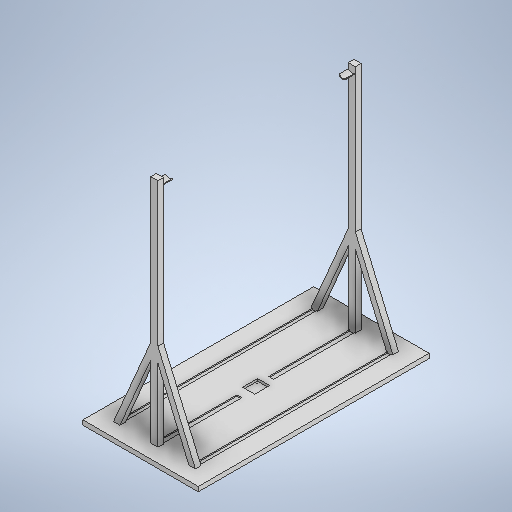
# Autodesk Inventor part: Structure_provisional
Saved by Autodesk Inventor 2025.1 (Build 291241020, 241B)
## iProperties
Created: 2025-09-05
Part Number: Structure_provisional
Material: Genérico
Document SubType Name: Modeling
Designer: Yo
Density: 1 g/cm^3
Appearance: Valor por defecto
Author: Yo
Autodesk Inventor part; units mm, degrees
ref_plane "YZ Plane" through (0, 0, 0) normal (1, 0, 0) x (0, 1, 0)
ref_plane "XZ Plane" through (0, 0, 0) normal (0, 1, 0) x (-1, 0, 0)
sketch "Boceto1" plane through (0, 0, 0) normal (0, 1, 0) x (-1, 0, 0)
  line L0 (0, 0) -> (0, -500) construction
  line L1 (0, -500) -> (500, -500) construction
  line L2 (500, -500) -> (500, 500) construction
  line L3 (500, 500) -> (0, 500) construction
  line L4 (0, 500) -> (0, 0) construction
  line L5 (500, 500) -> (0, 500)
  line L6 (0, 500) -> (0, -500)
  line L7 (0, -500) -> (500, -500)
  line L8 (500, -500) -> (500, 500)
  dimension "d0" = 500
  dimension "d1" = 500
  dimension "d2" = 1000
  constraints: 18 end point, 4 perpendicular, 3 equal length, 1 horizontal, 1 point on line, 1 vertical
  measures "d0" distance of L0.start L0.end
  measures "d1" distance of L0.end L1.end
  measures "d2" distance of L1.end L2.end
extrude "Extrusión1" add sketch "Boceto1" along normal blind 20
sketch "Boceto2" plane through (0, 20, 0) normal (0, 1, 0) x (1, 0, 0)
  line L0 (0, 500) -> (-500, 500) construction
  line L1 (-250, 500) -> (-250, -500) construction
  line L2 (-500, -500) -> (0, -500) construction
  line L3 (-265.9292, 440.1456) -> (-234.905, 440.1456)
  line L4 (-234.905, 440.1456) -> (-234.905, 415.7448)
  line L5 (-234.905, 415.7448) -> (-265.9292, 415.7448)
  line L6 (-265.9292, 415.7448) -> (-265.9292, 440.1456)
  point P0 (0, 0)
  constraints: 10 end point, 2 midpoint, 2 parallel, 1 horizontal, 1 perpendicular
extrude "Extrusión2" add sketch "Boceto2" along normal blind 1000
mirror "Simetría1" about plane through (0, 0, 0) normal (0, 0, 1) of "Extrusión2"
sketch "Boceto4" plane through (-265.9292, 20, 440.1456) normal (0, 0, 1) x (1, 0, 0)
  line L0 (31.0242, 0) -> (31.0242, 1000) construction
  line L1 (31.0242, 379.2693) -> (193.3148, 0) construction
  line L2 (31.0242, 314.0177) -> (165.3935, 0) construction
  line L3 (-234.0708, 0) -> (265.9292, 0) construction
  line L4 (31.0242, 379.2693) -> (193.3148, 0)
  line L5 (165.3935, 0) -> (31.0242, 314.0177)
  line L6 (31.0242, 379.2693) -> (31.0242, 314.0177)
  line L7 (165.3935, 0) -> (193.3148, 0)
  point P0 (265.9292, -20)
  constraints: 12 end point, 4 point on line, 3 collinear, 1 parallel
extrude "Extrusión3" add sketch "Boceto4" against normal up to surface (24.4008 mm away)
ref_plane "Plano de trabajo1" through (-250, 0, 500) normal (1, 0, 0) x (0, 0, -1)
mirror "Simetría2" about plane through (-250, 0, 500) normal (1, 0, 0) of "Extrusión3"
mirror "Simetría3" about plane through (0, 0, 0) normal (0, 0, 1) of "Extrusión3", "Simetría2"
sketch "Boceto5" plane through (0, 20, 0) normal (0, 1, 0) x (1, 0, 0)
  line L0 (-72.6144, 415.7448) -> (-234.905, 415.7448) construction
  line L1 (-78.0914, 415.7448) -> (-78.0914, 405.899) construction
  line L2 (-95.8718, 415.7448) -> (-95.8718, 405.899) construction
  line L3 (-78.0914, 415.7448) -> (-95.8718, 415.7448)
  line L4 (-95.8718, 0) -> (-95.8718, 415.7448)
  line L5 (-78.0914, 415.7448) -> (-78.0914, 0)
  line L6 (-78.0914, 0) -> (-78.0914, -415.7448)
  line L7 (-100.5357, -415.7448) -> (-72.6144, -415.7448) projected
  line L8 (-95.8718, 0) -> (-95.8718, -415.7448)
  line L9 (-78.0914, -415.7448) -> (-95.8718, -415.7448)
  point P0 (0, 0)
  constraints: 16 end point, 8 point on line, 2 collinear, 2 perpendicular, 1 vertical
extrude "Extrusión4" cut sketch "Boceto5" against normal blind 5
mirror "Simetría4" about plane through (-250, 0, 500) normal (1, 0, 0) of "Extrusión4"
sketch "Boceto6" plane through (0, 20, 0) normal (0, 1, 0) x (1, 0, 0)
  line L0 (-265.9292, 415.7448) -> (-234.905, 415.7448) construction
  line L1 (-239.0903, 415.7448) -> (-239.0903, 391.5107) construction
  line L2 (-260.3339, 415.7448) -> (-260.3339, 390.2687) construction
  line L3 (-265.9292, -415.7448) -> (-234.905, -415.7448) construction
  line L4 (-239.0903, 415.7448) -> (-260.3339, 415.7448) construction
  line L5 (-260.3339, -415.7448) -> (-239.0903, -415.7448) construction
  line L6 (-239.0903, -415.7448) -> (-260.3339, -415.7448)
  line L7 (-239.0903, 415.7448) -> (-260.3339, 415.7448)
  line L8 (-239.0903, 65.2159) -> (-260.3339, 65.2159)
  line L9 (-239.0903, -72.6288) -> (-260.3339, -72.6288)
  line L10 (-239.0903, -415.7448) -> (-239.0903, -72.6288)
  line L11 (-239.0903, 65.2159) -> (-239.0903, 415.7448)
  line L12 (-260.3339, 415.7448) -> (-260.3339, 65.2159)
  line L13 (-260.3339, -72.6288) -> (-260.3339, -415.7448)
  point P0 (0, 0)
  constraints: 24 end point, 6 perpendicular, 5 parallel, 3 point on line, 2 horizontal, 2 vertical, 1 collinear
extrude "Extrusión5" cut sketch "Boceto6" against normal blind 5
sketch "Boceto7" plane through (0, 20, 0) normal (0, 1, 0) x (1, 0, 0)
  line L0 (-224.1946, 33.7447) -> (-276.8566, 33.7447)
  line L1 (-276.8566, 33.7447) -> (-276.8566, -31.5828)
  line L2 (-276.8566, -31.5828) -> (-224.1946, -31.5828)
  line L3 (-224.1946, -31.5828) -> (-224.1946, 33.7447)
  point P0 (0, 0)
  constraints: 8 end point, 2 parallel, 1 horizontal, 1 perpendicular
extrude "Extrusión6" cut sketch "Boceto7" against normal blind 10
sketch "Boceto8" plane through (0, 10, 0) normal (0, 1, 0) x (1, 0, 0)
  point P0 (0, 0)
  point P1 (-230.6615, -24.5924)
hole "Agujero1" at (-230.6615, 10, 24.5924) direction (0, -1, 0) diameter 3 end through all
mirror "Simetría5" about plane through (-250, 0, 500) normal (1, 0, 0) of "Agujero1"
mirror "Simetría6" about plane through (0, 0, 0) normal (0, 0, 1) of "Agujero1", "Simetría5"
sketch "Boceto9" plane through (-265.9292, 397.3198, -415.7448) normal (0, 0, 1) x (1, 0, 0)
  line L0 (0, 0) -> (0, 622.6802) projected
  line L1 (31.0242, 1.9495) -> (31.0242, 622.6802) projected
  arc A0 (0, 595.7054) -> (31.0242, 595.8449) centre (15.4643, 606.4176) ccw
  line L2 (0, 595.7054) -> (0, 599.8174)
  line L3 (31.0242, 595.8449) -> (31.0242, 599.8174)
  arc A1 (0, 599.8174) -> (31.0242, 599.8174) centre (15.5121, 611.2009) ccw
  point P0 (265.9292, -397.3198)
  constraints: 4 end point, 4 point on circle, 4 point on line, 2 centre point
extrude "Extrusión7" add sketch "Boceto9" along normal blind 40
mirror "Simetría7" about plane through (0, 0, 0) normal (0, 0, 1) of "Extrusión7"
